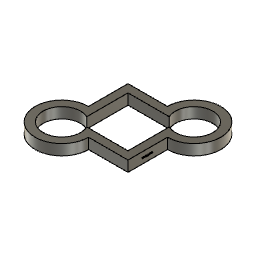
Model 26 (Autodesk Fusion 360 design; units mm, degrees)
Autodesk Fusion 360 part; units mm, degrees
sketch "Sketch1" plane through (0, 0, 0) normal (0, 0, 1) x (1, 0, 0)
  line L0 (47, -47) -> (-30.3772, -47)
  line L1 (-47, -30.3772) -> (-47, 47)
  line L2 (-47, 47) -> (30.3772, 47)
  line L3 (47, -47) -> (-47, 47) construction
  line L4 (-47, -47) -> (47, 47) construction
  line L5 (62, -62) -> (-12, -62)
  line L6 (62, 12) -> (62, -62)
  arc A0 (62, 12) -> (12, 62) centre (62, 62) ccw
  arc A1 (47, 30.3772) -> (30.3772, 47) centre (62, 62) ccw
  line L7 (-62, 62) -> (12, 62)
  line L8 (47, 30.3772) -> (47, -47)
  line L9 (-62, -12) -> (-62, 62)
  arc A2 (-62, -12) -> (-12, -62) centre (-62, -62) ccw
  arc A3 (-47, -30.3772) -> (-30.3772, -47) centre (-62, -62) ccw
  dimension "d1" = 94
  dimension "d2" = 94
  dimension "d4" = 70
  dimension "d5" = 100
  dimension "d6" = 70
  dimension "d7" = 100
  constraint horizontal L0
  constraint perpendicular L0 L1
  constraint parallel L0 L2
  constraint coincident L3 origin
  constraint coincident L4 origin
  constraint concentric A2 A3
  constraint concentric A0 A1
  constraint parallel L0 L5
  constraint parallel L2 L7
  measures "d1" distance of L1.end L4.end
  measures "d2" distance of L4.start L1.end
  measures "d4" diameter of A3
  measures "d5" diameter of A2
  measures "d6" diameter of A1
  measures "d7" diameter of A0
extrude "Extrude1" add sketch "Sketch1" along normal blind 20
ref_plane "WorkPlane1" through (62, -25, 10) normal (1, 0, 0) x (0, 1, 0)
sketch "Sketch2" plane through (62, -25, 10) normal (1, 0, 0) x (0, 1, 0)
  line L0 (-33.6097, -7.7243) -> (32.0106, -7.7243) construction
  line L1 (32.0106, -7.7243) -> (32.0106, 8.4783) construction
  line L2 (32.0106, 8.4783) -> (-33.6097, 8.4783) construction
  line L3 (-33.6097, 8.4783) -> (-33.6097, -7.7243) construction
  text T0 "enes şahin" font "Arial" height 3 align centre middle in box 65.6203 x 16.2025 at (-33.6097, -7.7243) x (1, 0) y (0, 1) spacing 1
extrude "Extrude2" add sketch "Sketch2" along normal blind 0.5 text T0
